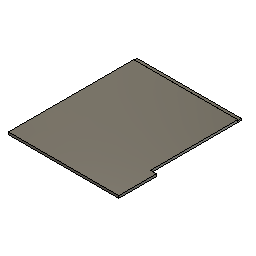
oceaan-25-floor_5 v2 (Autodesk Fusion 360 design; units mm, degrees)
Autodesk Fusion 360 part; units mm, degrees
sketch "Sketch1" plane through (0, 0, 0) normal (0, 1, 0) x (1, 0, 0)
  line L0 (5, 0) -> (5, 633)
  line L1 (571, 0) -> (571, 184)
  line L2 (539, 633) -> (539, 200)
  line L3 (571, 184) -> (540, 184)
  line L4 (539, 200) -> (539, 184)
  line L5 (539, 184) -> (540, 184)
  line L6 (5, 633) -> (5, 651)
  line L7 (539, 633) -> (539, 651)
  line L8 (539, 651) -> (5, 651)
  line L9 (5, 651) -> (5, 623)
  line L10 (539, 651) -> (539, 623)
  line L11 (5, 0) -> (5, -10)
  line L12 (571, 0) -> (571, -10)
  line L13 (571, -10) -> (5, -10)
  line L14 (5, 633) -> (539, 633)
  dimension "d1" = 633
  dimension "d3" = 184
  dimension "d4" = 534
  dimension "d5" = 433
  dimension "d6" = 31
  dimension "d7" = 16
  dimension "d8" = 18
  dimension "d9" = 18
  dimension "d10" = 28
  dimension "d11" = 28
  dimension "d12" = 10
  dimension "d13" = 10
  dimension "d14" = 566
  constraint vertical L0
  constraint perpendicular L1 L3
  constraint perpendicular L3 L4
  constraint vertical L7
  constraint coincident L2 L10.end
  constraint perpendicular L12 L13
  constraint perpendicular L7 L14
  constraint perpendicular L0 L13
  measures "d1" distance of L0.start L0.end
  measures "d3" distance of L1.start L1.end
  measures "d4" distance of L0.end L2.start
  measures "d5" distance of L2.start L2.end
  measures "d6" distance of L1.end L3.end
  measures "d7" distance of L2.end L4.end
  measures "d8" distance of L0.end L6.end
  measures "d9" distance of L2.start L7.end
  measures "d10" distance of L6.end L9.end
  measures "d11" distance of L7.end L10.end
  measures "d12" distance of L0.start L11.end
  measures "d13" distance of L1.start L12.end
  measures "d14" distance of L12.end L11.end
sketch "Sketch2" plane through (0, 0, 0) normal (0, 1, 0) x (1, 0, 0)
  line L0 (539, 633) -> (539, 200)
  line L1 (5, 633) -> (539, 633)
  line L2 (539, 633) -> (540, 184)
  line L3 (571, 184) -> (540, 184)
  line L4 (540, 184) -> (571, 184)
  line L5 (571, 184) -> (571, -10)
  line L6 (571, -10) -> (5, -10)
  line L7 (5, -10) -> (5, 633)
  point P0 (5, 633)
  point P1 (539, 633)
  point P2 (540, 184)
  point P3 (571, 184)
  point P4 (571, -10)
  point P5 (5, -10)
  constraint coincident P0 L1.start
  constraint coincident P1 L0.start
  constraint coincident P2 L2.end
  constraint coincident P3 L3.start
  constraint coincident P4 L5.end
  constraint coincident P5 L6.end
extrude "Extrude1" add sketch "Sketch1" sketch "Sketch2" against normal blind 9 contours L6 L7 L8 L9 L10 L14 of sketch 2
extrude "Extrude2" add sketch "Sketch2" along normal blind 3.5
